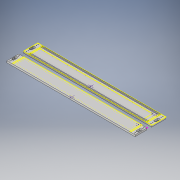
# Autodesk Inventor part: Button Fixture Base
Saved by Autodesk Inventor 2018 (Build 220112000, 112)
## iProperties
Created: 2016-07-07
Part Number: Button Fixture Base
Material: Generic
Document SubType Name: Modeling
Designer: Sam Clay
Density: 1 g/cm^3
Appearance: Default
Author: Sam Clay
Autodesk Inventor part; units mm, degrees
ref_plane "YZ Plane" through (0, 0, 0) normal (1, 0, 0) x (0, 1, 0)
ref_plane "XZ Plane" through (0, 0, 0) normal (0, 1, 0) x (-1, 0, 0)
ref_plane "XY Plane" through (0, 0, 0) normal (0, 0, 1) x (1, 0, 0)
sketch "Base Sketch" plane through (0, 0, 0) normal (0, 1, 0) x (-1, 0, 0)
  line L0 (0, 0) -> (1270, 0)
  line L1 (1270, 0) -> (1270, 152.4)
  line L2 (1270, 152.4) -> (0, 152.4)
  line L3 (0, 152.4) -> (0, 0)
  line L4 (1270, 0) -> (1320.8, 0)
  line L5 (1320.8, 0) -> (1320.8, 152.4)
  line L6 (1320.8, 152.4) -> (1270, 152.4)
  line L7 (1270, 152.4) -> (1270, 0)
  line L8 (0, 0) -> (-50.8, 0)
  line L9 (-50.8, 0) -> (-50.8, 152.4)
  line L10 (-50.8, 152.4) -> (0, 152.4)
  line L11 (0, 152.4) -> (0, 0)
  line L12 (1320.8, 152.4) -> (-50.8, 152.4)
  line L13 (-50.8, 152.4) -> (-50.8, 203.2)
  line L14 (-50.8, 203.2) -> (1320.8, 203.2)
  line L15 (1320.8, 203.2) -> (1320.8, 152.4)
  line L16 (-50.8, 203.2) -> (1320.8, 203.2)
  line L17 (1320.8, 203.2) -> (1320.8, 330.2)
  line L18 (1320.8, 330.2) -> (-50.8, 330.2)
  line L19 (-50.8, 330.2) -> (-50.8, 203.2)
  line L20 (1270, 203.2) -> (1270, 330.2)
  line L21 (0, 203.2) -> (0, 330.2)
  line L22 (1257.3, 152.4) -> (1257.3, 0)
  line L23 (12.7, 0) -> (12.7, 152.4)
  line L24 (12.7, 203.2) -> (12.7, 330.2)
  line L25 (1257.3, 203.2) -> (1257.3, 330.2)
  line L26 (1238.25, 222.25) -> (31.75, 222.25) construction
  line L27 (31.75, 222.25) -> (31.75, 311.15) construction
  line L28 (31.75, 311.15) -> (1238.25, 311.15) construction
  line L29 (1238.25, 311.15) -> (1238.25, 222.25) construction
  dimension "d0" = 1270
  dimension "d1" = 152.4
  dimension "d2" = 50.8
  dimension "d3" = 50.8
  dimension "d79" = 50.8
  dimension "d80" = 127
  dimension "d81" = 12.7
  dimension "d82" = 12.7
  dimension "d83" = 50.8
  dimension "d84" = 50.8
  dimension "d85" = 19.05
  dimension "d86" = 19.05
  dimension "d87" = 19.05
  dimension "d88" = 19.05
  constraints: 60 end point, 19 point on line, 12 parallel, 10 perpendicular, 6 horizontal
  measures "d0" distance of L2.end L1.end
  measures "d1" distance of L1.end L0.end
  measures "d2" distance of L6.end L5.end
  measures "d3" distance of L9.end L10.end
  measures "d79" distance of L9.end L13.end
  measures "d80" distance of L17.end L16.end
  measures "d81" distance between parallel lines of L22 L1
  measures "d82" distance between parallel lines of L23 L3
  measures "d83" distance between parallel lines of L19 L21
  measures "d84" distance between parallel lines of L17 L20
  measures "d85" distance between parallel lines of L26 L14
  measures "d86" distance between parallel lines of L25 L29
  measures "d87" distance between parallel lines of L24 L27
  measures "d88" distance between parallel lines of L18 L28
extrude "Base" add sketch "Base Sketch" along normal blind 19.05 contours L3 L2 L23 L0 | L23 L2 L22 L0 | L22 L2 L1 L0 | L21 L18 L24 L14 | L24 L18 L25 L14 | L25 L18 L20 L14
extrude "Lower Level" add sketch "Base Sketch" along normal blind 17.78 contours L8 L9 L10 L3 | L1 L6 L5 L4 | L19 L18 L21 L14 | L14 L20 L18 L17
sketch "Track Sketch" plane through (0, 19.05, 0) normal (0, 1, 0) x (1, 0, 0)
  line L0 (0, 0) -> (-1270, 0) projected
  line L1 (-1270, 0) -> (-1270, -152.4) projected
  line L2 (-1270, -152.4) -> (0, -152.4) projected
  line L3 (0, -152.4) -> (0, 0) projected
  line L4 (-1270, -3.175) -> (0, -3.175)
  line L5 (0, -152.4) -> (0, 0) projected
  line L6 (0, -22.987) -> (-1270, -22.987)
  line L7 (-1270, 0) -> (-1270, -152.4) projected
  line L8 (-1270, -149.225) -> (0, -149.225)
  line L9 (-1270, -129.413) -> (0, -129.413)
  line L10 (-50.8, -40.767) -> (-1270, -40.767)
  line L11 (-1270, -40.767) -> (-1270, -129.413)
  line L12 (-1270, -129.413) -> (-50.8, -129.413)
  line L13 (-50.8, -129.413) -> (-50.8, -40.767)
  circle A0 centre (-55.88, -45.847) radius 8.89
  dimension "d91" = 3.175
  dimension "d92" = 19.812
  dimension "d93" = 17.78
  dimension "d94" = 50.8
  dimension "d95" = 3.175
  dimension "d96" = 19.812
  dimension "d97" = 17.78
  dimension "d98" = 5.08
  dimension "d99" = 5.08
  constraints: 16 end point, 8 point on line, 4 perpendicular, 2 horizontal, 2 parallel, 1 centre point
  measures "d91" distance between parallel lines of L4 L0
  measures "d92" distance between parallel lines of L6 L4
  measures "d93" distance between parallel lines of L6 L10
  measures "d94" distance between parallel lines of L3 L13
  measures "d95" distance between parallel lines of L2 L8
  measures "d96" distance between parallel lines of L12 L8
  measures "d97" diameter of A0
  measures "d98" distance from line of L13 A0.centre
  measures "d99" distance from line of A0.centre L10
extrude "Tracks Cut" cut sketch "Track Sketch" against normal blind 11.43 contours L3 L6 L1 L4 | L3 L8 L1 L9
extrude "Pocket Side" cut sketch "Track Sketch" against normal blind 3.175 contours L10 A0 L13 L9 L1 | A0 L13 L10 | L10 L13 A0
sketch "Origin Sketch" plane through (0, 19.05, 0) normal (0, 1, 0) x (1, 0, 0)
  line L0 (50.8, 0) -> (-1320.8, 0) projected
  line L1 (50.8, -152.4) -> (50.8, 0) projected
  line L2 (-1320.8, -152.4) -> (50.8, -152.4) projected
  line L3 (-1320.8, 0) -> (-1320.8, -152.4) projected
  line L4 (0, -152.4) -> (0, -149.225) projected
  line L5 (0, -152.4) -> (50.8, -152.4) projected
  line L6 (50.8, -152.4) -> (50.8, 0) projected
  line L7 (50.8, 0) -> (0, 0) projected
  line L8 (0, -3.175) -> (0, 0) projected
  line L9 (0, -22.987) -> (0, -3.175) projected
  line L10 (0, -129.413) -> (0, -22.987) projected
  line L11 (0, -149.225) -> (0, -129.413) projected
  line L12 (-1270, -40.767) -> (-63.1756, -40.767) projected
  line L13 (0, -203.2) -> (-1270, -203.2) projected
  line L14 (0, -330.2) -> (0, -203.2) projected
  line L15 (-1238.25, -222.25) -> (-31.75, -222.25) construction
  line L16 (-1238.25, -311.15) -> (-1238.25, -222.25) construction
  line L17 (-31.75, -311.15) -> (-1238.25, -311.15) construction
  line L18 (-31.75, -222.25) -> (-31.75, -311.15) construction
  line L19 (-12.7, -203.2) -> (-12.7, -330.2) projected
  line L20 (0, -203.2) -> (0, -330.2) projected
  line L21 (-1270, -203.2) -> (-1270, -330.2) projected
  line L22 (-1257.3, -203.2) -> (-1257.3, -330.2) projected
  line L23 (-1257.3, -152.4) -> (-1257.3, 0) projected
  line L24 (-1270, 0) -> (-1270, -152.4) projected
  line L25 (-12.7, 0) -> (-12.7, -152.4) projected
  line L26 (0, -152.4) -> (0, 0) projected
  line L27 (-50.8, -53.1426) -> (-50.8, -129.413) projected
  point P0 (-25.4, -40.767)
  point P1 (50.8, -203.2)
  point P2 (-635, -116.967)
  point P3 (-25.4, -215.9)
  point P4 (-635, -317.5)
  dimension "d72" = 76.2
  dimension "d73" = 609.6
  dimension "d100" = 25.4
  dimension "d102" = 12.7
  dimension "d103" = 25.4
  dimension "d127" = 101.6
  dimension "d128" = 609.6
  constraints: 1 point on line, 1 other
  measures "d72" vertical distance of point (-635, -116.967) point (-25.4, -40.767)
  measures "d73" horizontal distance of point (-635, -116.967) point (-25.4, -40.767)
  measures "d100" distance from line of L10 point (-25.4, -40.767)
  measures "d102" distance from line of point (-25.4, -215.9) L13
  measures "d103" distance from line of L14 point (-25.4, -215.9)
  measures "d127" vertical distance of point (-635, -317.5) point (-25.4, -215.9)
  measures "d128" horizontal distance of point (-635, -317.5) point (-25.4, -215.9)
sketch "Handles Sketch" plane through (0, 17.78, 0) normal (0, 1, 0) x (1, 0, 0)
  line L0 (-1301.75, -47.625) -> (-1301.75, -104.775) construction
  line L1 (-1314.45, -60.325) -> (-1314.45, -92.075)
  line L2 (-1289.05, -92.075) -> (-1289.05, -60.325)
  arc A0 (-1289.05, -60.325) -> (-1314.45, -60.325) centre (-1301.75, -60.325) ccw
  arc A1 (-1314.45, -92.075) -> (-1289.05, -92.075) centre (-1301.75, -92.075) ccw
  line L3 (-1270, 0) -> (-1320.8, 0) projected
  line L4 (-1320.8, 0) -> (-1320.8, -152.4) projected
  line L5 (50.8, -152.4) -> (50.8, 0) projected
  line L6 (-1320.8, -152.4) -> (-1270, -152.4) projected
  line L7 (-1270, -203.2) -> (-1320.8, -203.2) projected
  line L8 (-1320.8, -330.2) -> (-1270, -330.2) projected
  line L9 (-1301.75, -241.3) -> (-1301.75, -292.1) construction
  line L10 (-1314.45, -254) -> (-1314.45, -279.4)
  line L11 (-1289.05, -279.4) -> (-1289.05, -254)
  arc A2 (-1289.05, -254) -> (-1314.45, -254) centre (-1301.75, -254) ccw
  arc A3 (-1314.45, -279.4) -> (-1289.05, -279.4) centre (-1301.75, -279.4) ccw
  line L12 (31.75, -47.625) -> (31.75, -104.775) construction
  line L13 (19.05, -60.325) -> (19.05, -92.075)
  line L14 (44.45, -92.075) -> (44.45, -60.325)
  arc A4 (44.45, -60.325) -> (19.05, -60.325) centre (31.75, -60.325) ccw
  arc A5 (19.05, -92.075) -> (44.45, -92.075) centre (31.75, -92.075) ccw
  line L15 (31.75, -241.3) -> (31.75, -292.1) construction
  line L16 (19.05, -254) -> (19.05, -279.4)
  line L17 (44.45, -279.4) -> (44.45, -254)
  arc A6 (44.45, -254) -> (19.05, -254) centre (31.75, -254) ccw
  arc A7 (19.05, -279.4) -> (44.45, -279.4) centre (31.75, -279.4) ccw
  point P0 (0, 0)
  point P1 (31.75, -12.7)
  point P2 (31.75, -31.75)
  point P3 (31.75, -120.65)
  point P4 (31.75, -139.7)
  point P5 (31.75, -215.9)
  point P6 (31.75, -228.6)
  point P7 (31.75, -304.8)
  point P8 (31.75, -317.5)
  point P9 (-1301.75, -317.5)
  point P10 (-1301.75, -304.8)
  point P11 (-1301.75, -228.6)
  point P12 (-1301.75, -215.9)
  point P13 (-1301.75, -139.7)
  point P14 (-1301.75, -120.65)
  point P15 (-1301.75, -31.75)
  point P16 (-1301.75, -12.7)
  point P17 (-1301.75, -76.2)
  point P18 (-1301.75, -266.7)
  point P19 (31.75, -76.2)
  point P20 (31.75, -266.7)
  dimension "d104" = 57.15
  dimension "d105" = 25.4
  dimension "d106" = 76.2
  dimension "d107" = 19.05
  dimension "d108" = 19.05
  dimension "d109" = 19.05
  dimension "d110" = 12.7
  dimension "d111" = 19.05
  dimension "d112" = 12.7
  dimension "d113" = 19.05
  dimension "d114" = 12.7
  dimension "d115" = 12.7
  dimension "d116" = 12.7
  dimension "d117" = 12.7
  dimension "d118" = 50.8
  dimension "d119" = 25.4
  dimension "d120" = 63.5
  dimension "d121" = 57.15
  dimension "d122" = 25.4
  dimension "d123" = 50.8
  dimension "d124" = 25.4
  constraints: 32 end point, 24 point on circle, 17 vertical alignment, 16 tangent, 10 horizontal alignment, 10 point on line, 8 centre point, 4 midpoint, 4 parallel, 3 vertical
  measures "d104" distance of L0.start L0.end
  measures "d105" diameter of A1
  measures "d106" distance from line of point (-1301.75, -76.2) L3
  measures "d107" distance from line of L4 point (-1301.75, -76.2)
  measures "d108" distance from line of L4 point (-1301.75, -12.7)
  measures "d109" distance from line of point (31.75, -12.7) L5
  measures "d110" distance from line of L3 point (-1301.75, -12.7)
  measures "d111" distance of point (-1301.75, -12.7) point (-1301.75, -31.75)
  measures "d112" distance from line of L6 point (-1301.75, -139.7)
  measures "d113" distance of point (-1301.75, -120.65) point (-1301.75, -139.7)
  measures "d114" distance from line of point (-1301.75, -215.9) L7
  measures "d115" distance of point (-1301.75, -215.9) point (-1301.75, -228.6)
  measures "d116" distance from line of L8 point (-1301.75, -317.5)
  measures "d117" distance of point (-1301.75, -304.8) point (-1301.75, -317.5)
  measures "d118" distance of L9.start L9.end
  measures "d119" diameter of A3
  measures "d120" distance from line of point (-1301.75, -266.7) L7
  measures "d121" distance of L12.start L12.end
  measures "d122" diameter of A5
  measures "d123" distance of L15.start L15.end
  measures "d124" diameter of A7
extrude "Extrusion6" cut sketch "Handles Sketch" against normal through all
hole "Hole1" at (-25.4, 19.05, 40.767) at (-635, 19.05, 317.5) at (-25.4, 19.05, 215.9) direction (0, -1, 0) diameter 3.175 depth 1.27
hole "Hole3" at (-635, 19.05, 116.967) direction (0, -1, 0) diameter 3.175 depth 4.445 tip angle 118
hole "Hole2" at (-1301.75, 17.78, 12.7) at (-1301.75, 17.78, 31.75) at (-1301.75, 17.78, 120.65) at (-1301.75, 17.78, 139.7) at (-1301.75, 17.78, 215.9) at (-1301.75, 17.78, 228.6) at (-1301.75, 17.78, 304.8) at (-1301.75, 17.78, 317.5) at (31.75, 17.78, 215.9) at (31.75, 17.78, 228.6) at (31.75, 17.78, 304.8) at (31.75, 17.78, 317.5) at (31.75, 17.78, 139.7) at (31.75, 17.78, 120.65) at (31.75, 17.78, 31.75) at (31.75, 17.78, 12.7) direction (0, -1, 0) diameter 6.35 end through all
body "Solid1"
